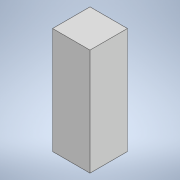
# Autodesk Inventor part: latticeStandIn
Saved by Autodesk Inventor 2020.5 (Build 245400000, 400)
## iProperties
Created: 2022-09-15
Part Number: latticeStandIn
Material: Generic
Document SubType Name: Modeling
Designer: kouda
Density: 1 g/cm^3
Appearance: Default
Author: kouda
Autodesk Inventor part; units mm, degrees
ref_plane "YZ Plane" through (0, 0, 0) normal (1, 0, 0) x (0, 1, 0)
ref_plane "XZ Plane" through (0, 0, 0) normal (0, 1, 0) x (-1, 0, 0)
ref_plane "XY Plane" through (0, 0, 0) normal (0, 0, 1) x (1, 0, 0)
sketch "Sketch1" plane through (0, 0, 0) normal (0, 1, 0) x (-1, 0, 0)
  line L0 (0, 0) -> (6.5, 0)
  line L1 (6.5, 0) -> (6.5, -6.5)
  line L2 (6.5, -6.5) -> (0, -6.5)
  line L3 (0, -6.5) -> (0, 0)
  dimension "d0" = 6.5
  dimension "d1" = 6.5
  constraints: 8 end point, 2 parallel, 1 horizontal, 1 perpendicular
  measures "d0" distance of L1.end L2.end
  measures "d1" distance of L0.end L1.end
extrude "Extrusion1" add sketch "Sketch1" along normal blind 18.5
body "Solid1"
